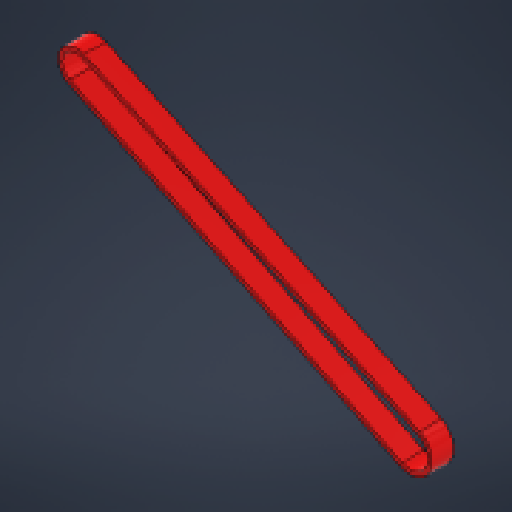
# Autodesk Inventor part: Single Indexer tensioner band
Saved by Autodesk Inventor 2023.2 (Build 272271030, 271C)
## iProperties
Created: 2023-04-07
Part Number: Single Indexer tensioner band
Material: Generic
Document SubType Name: Modeling
Designer: Main Account
Density: 1 g/cm^3
Appearance: Default
Author: Main Account
Autodesk Inventor part; units mm, degrees
ref_plane "YZ Plane" through (0, 0, 0) normal (1, 0, 0) x (0, 1, 0)
ref_plane "XZ Plane" through (0, 0, 0) normal (0, 1, 0) x (-1, 0, 0)
ref_plane "XY Plane" through (0, 0, 0) normal (0, 0, 1) x (1, 0, 0)
sketch "Sketch1" plane through (0, 0, 0) normal (0, 0, 1) x (1, 0, 0)
  circle A0 centre (0, 0) radius 4.064 construction
  circle A1 centre (-76.1973, 37.0416) radius 3.9624 construction
  arc A2 (-74.8392, 39.9115) -> (-77.6153, 34.2009) centre (-76.1973, 37.0416) ccw
  line L0 (-74.8392, 39.9115) -> (1.7384, 3.6735)
  line L1 (-1.8151, -3.6362) -> (-77.6153, 34.2009)
  arc A3 (-1.8151, -3.6362) -> (1.7384, 3.6735) centre (0, 0) ccw
  line L2 (2.1661, 4.5774) -> (-74.4115, 40.8154)
  arc A4 (-74.4115, 40.8154) -> (-78.0619, 33.3061) centre (-76.1973, 37.0416) ccw
  line L3 (-78.0619, 33.3061) -> (-2.2617, -4.5309)
  arc A5 (-2.2617, -4.5309) -> (2.1661, 4.5774) centre (0, 0) ccw
  point P0 (0, 0)
  dimension "d0" = 6.35
  dimension "d1" = 1
  constraints: 10 point on circle, 8 end point, 4 centre point, 2 coincident, 2 tangent, 1 concentric, 3 other
  measures "d0" diameter of A2
  measures "d1" distance between parallel lines of L0 L2
extrude "Extrusion1" add sketch "Sketch1" against normal blind 5
body "Solid1"
